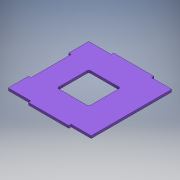
# Autodesk Inventor part: Control lateral
Saved by Autodesk Inventor 2018 (Build 220112000, 112)
## iProperties
Created: 2020-03-09
Part Number: Control lateral
Material: Genérico
Document SubType Name: Modeling
Designer: joser
Density: 1 g/cm^3
Appearance: Violeta
Author: joser
Autodesk Inventor part; units mm, degrees
ref_plane "YZ Plane" through (0, 0, 0) normal (1, 0, 0) x (0, 1, 0)
ref_plane "XZ Plane" through (0, 0, 0) normal (0, 1, 0) x (-1, 0, 0)
ref_plane "XY Plane" through (0, 0, 0) normal (0, 0, 1) x (1, 0, 0)
sketch "Boceto1" plane through (0, 0, 0) normal (0, 0, 1) x (1, 0, 0)
  line L0 (0, 100) -> (0, 0)
  line L1 (-100, 25) -> (-100, 75)
  line L2 (-75, 0) -> (-75, -3)
  line L3 (-75, -3) -> (-25, -3)
  line L4 (-25, -3) -> (-25, 0)
  line L5 (0, 0) -> (-25, 0)
  line L6 (-103, 100) -> (-103, 75)
  line L7 (-103, 75) -> (-100, 75)
  line L8 (-103, 0) -> (-103, 25)
  line L9 (-103, 25) -> (-100, 25)
  line L10 (-103, 0) -> (-75, 0)
  line L11 (-75, 100) -> (-75, 103)
  line L12 (-75, 103) -> (-25, 103)
  line L13 (-25, 103) -> (-25, 100)
  line L14 (0, 100) -> (-25, 100)
  line L15 (-75, 100) -> (-103, 100)
  dimension "d1" = 100
  dimension "d4" = 50
  dimension "d5" = 25
  dimension "d7" = 25
  dimension "d8" = 25
  dimension "d9" = 3
  dimension "d10" = 3
  dimension "d11" = 100
  dimension "d13" = 50
  dimension "d14" = 3
  constraints: 32 end point, 9 perpendicular, 4 collinear, 3 horizontal, 2 vertical, 1 coincident, 1 parallel
  measures "d1" distance of L0.start L0.end
  measures "d4" distance of L2.end L3.end
  measures "d5" distance between parallel lines of L0 L4
  measures "d7" distance of L6.start L6.end
  measures "d8" distance of L8.start L8.end
  measures "d9" distance between parallel lines of L1 L6
  measures "d10" distance between parallel lines of L10 L3
  measures "d11" distance between parallel lines of L0 L1
  measures "d13" distance of L11.end L12.end
  measures "d14" distance between parallel lines of L15 L12
extrude "Extrusión2" add sketch "Boceto1" along normal blind 3
sketch "Boceto2" plane through (0, 0, 3) normal (0, 0, 1) x (1, 0, 0)
  line L0 (-75, 100) -> (-103, 100) projected
  line L1 (-72.75, 69.75) -> (-33.25, 69.75)
  line L2 (-33.25, 69.75) -> (-33.25, 30.25)
  line L3 (-33.25, 30.25) -> (-72.75, 30.25)
  line L4 (-72.75, 30.25) -> (-72.75, 69.75)
  line L5 (-103, 25) -> (-103, 0) projected
  point P0 (0, 0)
  dimension "d37" = 39.5
  dimension "d38" = 39.5
  dimension "d39" = 30.25
  dimension "d40" = 30.25
  constraints: 8 end point, 2 parallel, 1 horizontal, 1 perpendicular
  measures "d37" distance of L2.end L3.end
  measures "d38" distance of L1.end L2.end
  measures "d39" distance between parallel lines of L1 L0
  measures "d40" distance between parallel lines of L4 L5
extrude "Extrusión3" cut sketch "Boceto2" against normal blind 3
fillet "Empalme1" radius 2 4 edges at (-72.75, 69.75, 1.5) (-33.25, 69.75, 1.5) (-33.25, 30.25, 1.5) (-72.75, 30.25, 1.5)
